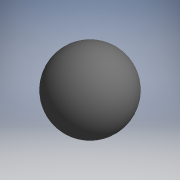
# Autodesk Inventor part: 684AZZ Ball
Saved by Autodesk Inventor 2017.3 (Build 213256000, 256)
## iProperties
Part Number: 684AZZ Ball
Material: Generic
Catalog Web Link: www.cadenas.de
Description: shielde_type_zz_zzs_B-
Vendor: NSK_RB
Document SubType Name: Modeling
Designer: partserver
Manufacturer: NSK_RB
Mass: 0.00176715 g
Surface Area: 0.0706858 cm^2
Volume: 0.00176715 cm^3
Density: 1 g/cm^3
Appearance: PSOLRGB-128-128-128
Category: PARTsolutions
Company: NSK_RB
Title: 684AZZ Ball
Author: Cadenas PARTsolutions
PSOL_IDENT_0: {$CADENAS_DATA\23d-libs\nsk_rb\roller_bearings\deep_groove_bb\exstra_small_miniatur_bb\metric_design
PSOL_IDENT_1: \shielded_type_zz_zzs_b.prj},178 {VTYP=3D},{NB=684AZZ Ball},{LINA=684AZZ Ball},{NN=shielde_type_zz_z
PSOL_IDENT_2: zs_B},{DATE=30.03.2022 01:55:07},{GEOMDATE=04.01.2008 00:00:00},{VERSION=},{LINEID=220},{WBVAR=},{WB
PSOL_IDENT_3: NUMERIC=}  {NB=684AZZ Ball},{LINA=684AZZ Ball},{KT=DUMMY},{IDNR=},{STAN=Standard},{ORDER=684AZZ},{SD=
PSOL_IDENT_4: 4.0},{X=4.0},{DI1=5.20},{DI2=5.20},{SDE1=7.50},{SDE2=8.10},{D=9},{DD=9},{B=0.0},{B1=4.0},{R=0.00},{R
PSOL_IDENT_5: 1=0.15},{CR1=640},{COR1=225},{CR2=65},{COR2=23.0},{LG=53000},{LO=63000},{DA=0.0},{DB=5.2},{DA1=0.0},
PSOL_IDENT_6: {DB1=8.1},{RA=0.00},{RB=0.10},{MASS=1.01},{SC=1}
NB: 684AZZ Ball
NN: shielde_type_zz_zzs_B
NBSYN: $ORDER. Ball
LINA: 684AZZ Ball
CATALOG: NSK Rolling Bearing
STAN: Standard
ORDER: 684AZZ
SD: 4
X: 4
DI1: 5.2
DI2: 5.2
SDE1: 7.5
SDE2: 8.1
D: 9
DD: 9
B: 0
B1: 4
R: 0
R1: 0.15
CR1: 640
COR1: 225
CR2: 65
COR2: 23
LG: 53000
LO: 63000
DA: 0
DB: 5.2
DA1: 0
DB1: 8.1
RA: 0
RB: 0.1
MASS: 1.01
SC: 1
SUPPLIER: NSK_RB
ARTICLENO: 684AZZ Ball
BOMINFO: 684AZZ Ball
CREATOR: CADENAS GmbH
Autodesk Inventor part; units mm, degrees
sketch "Sketch_1" plane through (0, 0, 0) normal (0, 0, 1) x (1, 0, 0)
  line L0 (0.75, 0) -> (-0.75, 0)
  arc A0 (0.75, 0) -> (-0.75, 0) centre (0, 0) ccw
  line L1 (0.75, 0) -> (-0.75, 0)
  constraints: 4 end point, 2 point on circle, 1 centre point
revolve "Revolution1" add sketch "Sketch_1" angle 360 about axis through (0.75, 0, 0) along (1, 0, 0)
ref_plane "ip_st_b_XY" through (0, 0, 0) normal (-1, 0, 0) x (0, 0, -1)
ref_plane "ip_st_b_YZ" through (0, 0, 0) normal (0, 0, -1) x (0, -1, 0)
ref_plane "ip_st_b_ZX" through (0, 0, 0) normal (0, -1, 0) x (-1, 0, 0)
body "Solid1"
